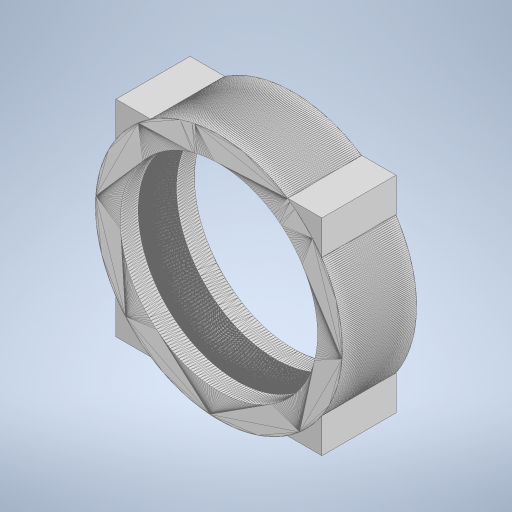
# Autodesk Inventor part: bearing-gairin
Saved by Autodesk Inventor 2024 (Build 280153000, 153)
## iProperties
Created: 2024-02-10
Part Number: bearing-gairin
Material: 一般
Document SubType Name: Modeling
Designer: mott1
Density: 1 g/cm^3
Appearance: 既定
Author: mott1
Autodesk Inventor part; units mm, degrees
ref_plane "YZ Plane" through (0, 0, 0) normal (1, 0, 0) x (0, 1, 0)
ref_plane "XZ Plane" through (0, 0, 0) normal (0, 1, 0) x (-1, 0, 0)
ref_plane "XY Plane" through (0, 0, 0) normal (0, 0, 1) x (1, 0, 0)
sketch "スケッチ1" plane through (8.3334, 12.4721, 4.5) normal (0, 0, 1) x (1, 0, 0)
  circle A0 centre (-8.3334, -12.4721) radius 15
  line L0 (4.1666, 0.0279) -> (-0.0418, 0.0279)
  line L1 (-16.625, 0.0279) -> (-20.8334, 0.0279)
  line L2 (-20.8334, 0.0279) -> (-20.8334, -4.1806)
  line L3 (-20.8334, -20.7637) -> (-20.8334, -24.9721)
  line L4 (-20.8334, -24.9721) -> (-16.625, -24.9721)
  line L5 (-0.0418, -24.9721) -> (4.1666, -24.9721)
  line L6 (4.1666, -24.9721) -> (4.1666, -20.7637)
  line L7 (4.1666, -4.1806) -> (4.1666, 0.0279)
  dimension "d4" = 30
  dimension "d2" = 25
  dimension "d3" = 25
  constraints: 16 end point, 8 parallel, 4 perpendicular, 2 horizontal, 1 coincident, 10 other
  measures "d2" distance of L5.end L3.end
  measures "d3" distance of L3.end L1.end
extrude "押し出し1" add sketch "スケッチ1" against normal blind 9 contours A0 L0 L7 | L6 L5 A0 | A0 L2 L1 | L4 L3 A0
